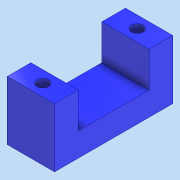
# Autodesk Inventor part: aux_axis_cap
Saved by Autodesk Inventor 2022 (Build 260153000, 153)
## iProperties
Created: 2021-08-09
Part Number: aux_axis_cap
Material: Generic
Document SubType Name: Modeling
Designer: nnico
Density: 1 g/cm^3
Appearance: Blue - Wall Paint - Glossy
Author: nnico
Autodesk Inventor part; units mm, degrees
ref_plane "YZ Plane" through (0, 0, 0) normal (1, 0, 0) x (0, 1, 0)
ref_plane "XZ Plane" through (0, 0, 0) normal (0, 1, 0) x (-1, 0, 0)
ref_plane "XY Plane" through (0, 0, 0) normal (0, 0, 1) x (1, 0, 0)
sketch "Sketch1" plane through (0, 0, 0) normal (1, 0, 0) x (0, 1, 0)
  line L0 (15, 15) -> (0, 15)
  line L1 (0, 15) -> (0, 0)
  line L2 (15, 15) -> (15, 0) construction
  line L3 (15, 15) -> (15, 25)
  line L4 (15, 25) -> (-10, 25)
  line L5 (-10, 25) -> (-10, 0)
  line L6 (-10, 0) -> (15, 0) construction
  line L7 (15, -15) -> (0, -15)
  line L8 (0, -15) -> (0, 0)
  line L9 (15, -15) -> (15, 0) construction
  line L10 (15, -15) -> (15, -25)
  line L11 (15, -25) -> (-10, -25)
  line L12 (-10, -25) -> (-10, 0)
  dimension "d0" = 15
  dimension "d1" = 15
  dimension "d2" = 10
  dimension "d3" = 25
  constraints: 26 end point, 4 symmetric about line, 3 perpendicular, 2 horizontal, 2 vertical, 1 coincident
  measures "d0" distance of L0.start L0.end
  measures "d1" distance of L0.end L1.end
  measures "d2" distance of L0.start L3.end
  measures "d3" distance of L3.end L4.end
extrude "Extrusion1" add sketch "Sketch1" along normal blind 20
sketch "Sketch2" plane through (0, 15, 25) normal (0, 1, 0) x (1, 0, 0)
  line L0 (0, 25) -> (20, 25) construction
  line L1 (20, 40) -> (20, 10) construction
  line L2 (20, 0) -> (20, 50) construction
  line L3 (0, 10) -> (20, 10) construction
  line L4 (20, 0) -> (0, 10) construction
  line L5 (0, 0) -> (20, 0) construction
  line L6 (0, 0) -> (20, 10) construction
  circle A0 centre (10, 5) radius 2.5
  circle A1 centre (10, 45) radius 2.5
  dimension "d6" = 5
  constraints: 6 end point, 2 centre point, 2 midpoint, 1 symmetric about line, 1 other
  measures "d6" diameter of A0
extrude "Extrusion2" cut sketch "Sketch2" against normal blind 4
body "Solid1"
